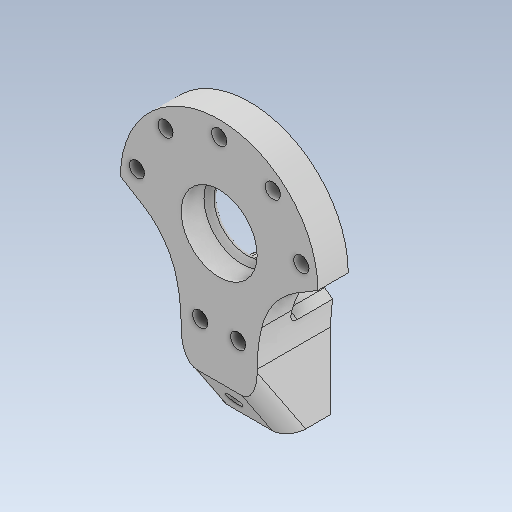
# Autodesk Inventor part: bone_upper_2
Saved by Autodesk Inventor 2020 (Build 240168000, 168)
## iProperties
Created: 2019-05-04
Part Number: bone_upper_2
Material: Generic
Document SubType Name: Modeling
Designer: psrob
Density: 1 g/cm^3
Appearance: Default
Author: psrob
Autodesk Inventor part; units mm, degrees
ref_plane "YZ Plane" through (0, 0, 0) normal (1, 0, 0) x (0, 1, 0)
ref_plane "XZ Plane" through (0, 0, 0) normal (0, 1, 0) x (-1, 0, 0)
ref_plane "XY Plane" through (0, 0, 0) normal (0, 0, 1) x (1, 0, 0)
sketch "Sketch1" plane through (0, 0, 0) normal (0, 0, 1) x (1, 0, 0)
  line L0 (0, 50) -> (6, 50) projected
  circle A0 centre (3, -17) radius 2 projected
  line L1 (3, -17) -> (3, 63)
  circle A1 centre (3, 63) radius 8
  line L2 (6, 50) -> (8, 50)
  line L3 (8, 50) -> (-2, 50)
  line L4 (-2, 50) -> (-2, 40)
  line L5 (-2, 40) -> (8, 40)
  line L6 (8, 40) -> (8, 50)
  line L7 (3, 63) -> (10.191, 59.4944)
  line L8 (3, 63) -> (-4.191, 59.4944)
  arc A2 (10.191, 59.4944) -> (8, 50) centre (29.6667, 50) ccw
  arc A3 (-2, 50) -> (-4.191, 59.4944) centre (-23.6667, 50) ccw
  arc A4 (10.191, 59.4944) -> (-4.191, 59.4944) centre (3, 63) ccw
  point P0 (0, 0)
  dimension "d0" = 80
  dimension "d1" = 16
  dimension "d2" = 2
  dimension "d3" = 10
  dimension "d4" = 10
  dimension "d5" = 8
  constraints: 16 end point, 8 point on circle, 4 centre point, 4 line through centre, 2 horizontal, 2 parallel, 1 coincident, 1 perpendicular, 1 vertical
  measures "d0" distance of L1.start L1.end
  measures "d1" diameter of A1
  measures "d2" distance of L0.end L2.end
  measures "d3" distance of L5.end L4.end
  measures "d4" distance of L4.end L3.end
  measures "d5" radius of A4
extrude "Extrusion1" add sketch "Sketch1" along normal blind 10 contours L3 A3 A1 L1 L0 | L0 L1 L5 L4 L3 | L1 A1 A2 L2 L0 | L0 L2 L6 L5 L1 | A1 L8 L1 | L1 L7 A1 | A1 L7 L8
sketch "Sketch2" plane through (0, 0, 0) normal (0, 0, -1) x (-1, 0, 0)
  arc A0 (4.191, 59.4944) -> (-10.191, 59.4944) centre (-3, 63) ccw projected
  arc A1 (-8, 50) -> (-10.191, 59.4944) centre (-29.6667, 50) ccw projected
  line L0 (-8, 40) -> (-8, 50) projected
  line L1 (2, 40) -> (-8, 40) projected
  line L2 (2, 50) -> (2, 40) projected
  arc A2 (4.191, 59.4944) -> (2, 50) centre (23.6667, 50) ccw projected
  circle A3 centre (-3, 63) radius 9
  point P0 (0, 0)
  dimension "d8" = 18
  constraints: 1 centre point, 1 coincident
  measures "d8" diameter of A3
extrude "Extrusion2" cut sketch "Sketch2" against normal blind 2.7 contours A2 A3 A1 A0 | A0 A1 A3 A2
sketch "Sketch3" plane through (0, 0, 0) normal (0, 0, -1) x (-1, 0, 0)
  arc A0 (-8.9096, 56.212) -> (2.9096, 56.212) centre (-3, 63) ccw projected
  arc A1 (-8, 50) -> (-8.9096, 56.212) centre (-29.6667, 50) ccw projected
  line L0 (-8, 40) -> (-8, 50) projected
  line L1 (2, 40) -> (-8, 40) projected
  line L2 (2, 50) -> (2, 40) projected
  arc A2 (2.9096, 56.212) -> (2, 50) centre (23.6667, 50) ccw projected
  line L3 (-6, 50) -> (0, 50) projected
  line L4 (0, 0) -> (0, 50) projected
  line L5 (-6, 0) -> (-6, 50) projected
  point P0 (-6, 40)
  point P1 (0, 40)
extrude "Extrusion3" add sketch "Sketch3" along normal blind 3 contours A0 A2 L2 L1 L4 L3 L5 L0 A1
chamfer "Chamfer1" distance 3 angle 45 4 edges at (8.9096, 56.212, -1.5) (8.9096, 56.212, 1.35) (-2.9096, 56.212, -1.5) (-2.9096, 56.212, 1.35)
fillet "Fillet1" radius 1 3 edges at (7.3004, 53.9661, 2.7) (3, 54, 2.7) (-1.3004, 53.9661, 2.7)
thicken "Thicken1" operation add thickness 3.3 both sides no extend neighbours yes toward (0, 0, -1) faces at (4.7662, 63.054, 10)
sketch "Sketch4" plane through (0, 0, -3) normal (0, 0, -1) x (-1, 0, 0)
  line L0 (0.3503, 54.6468) -> (2.2505, 53.2853) projected
  arc A0 (-6.3503, 54.6468) -> (0.3503, 54.6468) centre (-3, 63) ccw projected
  line L1 (-8.2505, 53.2853) -> (-6.3503, 54.6468) projected
  arc A1 (-8, 50) -> (-8.2505, 53.2853) centre (-29.6667, 50) ccw projected
  line L2 (-8, 50) -> (-8, 40) projected
  line L3 (-8, 40) -> (-6, 40) projected
  line L4 (-6, 40) -> (-6, 50) projected
  line L5 (-6, 50) -> (0, 50) projected
  line L6 (0, 50) -> (0, 40) projected
  line L7 (0, 40) -> (2, 40) projected
  line L8 (2, 40) -> (2, 50) projected
  arc A2 (2.2505, 53.2853) -> (2, 50) centre (23.6667, 50) ccw projected
  line L9 (-6, 50) -> (0, 50) projected
  line L10 (-3, 50) -> (-3, 52)
  line L11 (-3, 52) -> (-0.5, 52)
  line L12 (-0.5, 52) -> (-5.5, 52)
  circle A3 centre (-0.5, 52) radius 1
  circle A4 centre (-5.5, 52) radius 1
  point P0 (0, 0)
  dimension "d19" = 2
  dimension "d20" = 2.5
  dimension "d21" = 5
  dimension "d22" = 2
  dimension "d23" = 2
  constraints: 6 end point, 2 centre point, 2 coincident, 1 midpoint, 1 perpendicular, 1 point on line, 1 vertical
  measures "d19" distance of L10.start L10.end
  measures "d20" distance of L10.end L11.end
  measures "d21" distance of L11.end L12.end
  measures "d22" diameter of A3
  measures "d23" diameter of A4
extrude "Extrusion4" cut sketch "Sketch4" against normal blind 10 contours A3 | A4
sketch "Sketch5" plane through (8, 40, -3) normal (1, 0, 0) x (0, 0, -1)
  line L0 (0, 10) -> (-9.7, 10) projected
  line L1 (-9.7, 0) -> (-9.7, 10) projected
  line L2 (0, 0) -> (-9.7, 0) projected
  line L3 (0, 10) -> (0, 0) projected
  line L4 (-9.7, 0) -> (-9.7, 10) projected
  line L5 (-9.7, 0) -> (-9.7, 6)
  line L6 (-9.7, 0) -> (-5.7, 0)
  line L7 (0, 0) -> (-9.7, 0) projected
  line L8 (-9.7, 6) -> (-5.7, 0)
  point P0 (-3, -40)
  point P1 (-5.7, 0)
  dimension "d26" = 6
  dimension "d27" = 4
  constraints: 6 end point, 2 point on line
  measures "d26" distance of L1.start L5.end
  measures "d27" distance of L1.start L6.end
extrude "Extrusion5" cut sketch "Sketch5" against normal blind 10 contours L8 L2 L1
fillet "Fillet2" radius 2 2 edges at (-2, 43, 4.7) (8, 43, 4.7)
fillet "Fillet3" radius 2 6 edges at (6.3897, 54.9866, 2.4133) (6.3503, 54.6468, -1.5) (6.3503, 54.6468, 0.85) (-0.3897, 54.9863, 2.4131) (-0.3503, 54.6468, 0.85) (-0.3503, 54.6468, -1.5)
sketch "Sketch6" plane through (0, 46, 6.7) normal (0, -0.5547002, 0.8320503) x (1, 0, 0)
  line L0 (6, 0) -> (6, -7.2111) projected
  line L1 (0, 0) -> (6, 0) projected
  line L2 (0, -7.2111) -> (0, 0) projected
  line L3 (6, -7.2111) -> (0, -7.2111) projected
  line L4 (0, -7.2111) -> (6, 0)
  line L5 (6, -7.2111) -> (0, 0)
  circle A0 centre (3, -3.6056) radius 1
  point P0 (0, -41.9908)
  dimension "d32" = 2
  constraints: 4 end point, 1 centre point, 1 midpoint
  measures "d32" diameter of A0
extrude "Extrusion6" cut sketch "Sketch6" against normal blind 7 contours A0 L5 L4 | L4 L5 A0 | A0 L4 L5 | L5 L4 A0
sketch "Sketch7" plane through (3, 63, 6.7) normal (0, 0, 1) x (1, 0, 0)
  ellipse E0 centre (3, -13.3944) end of major axis (3, -17) minor radius 2 (3, -17) -> (5, -13.3944) ccw projected
  line L0 (5, -13.3944) -> (5, -13) projected
  arc A0 (7.191, -3.5056) -> (5, -13) centre (26.6667, -13) ccw projected
  arc A1 (7.191, -3.5056) -> (-7.191, -3.5056) centre (0, 0) ccw projected
  arc A2 (-5, -13) -> (-7.191, -3.5056) centre (-26.6667, -13) ccw projected
  line L1 (-5, -13) -> (-5, -13.3944) projected
  ellipse E1 centre (-3, -13.3944) end of major axis (-3, -17) minor radius 2 (-5, -13.3944) -> (-3, -17) ccw projected
  line L2 (-3, -17) -> (3, -17) projected
  circle A3 centre (-2.5, -11) radius 1 projected
  circle A4 centre (2.5, -11) radius 1 projected
  circle A5 centre (0, 0) radius 5
  point P0 (-3, -63)
  dimension "d35" = 10
  constraints: 1 centre point, 1 coincident, 2 other
  measures "d35" diameter of A5
extrude "Extrusion7" cut sketch "Sketch7" against normal blind 7 contours A5
sketch "Sketch8" plane through (0, 0, 2.7) normal (0, 0, -1) x (-1, 0, 0)
  circle A0 centre (-3, 63) radius 5 projected
  circle A1 centre (-3, 63) radius 4
  point P0 (0, 0)
  dimension "d38" = 8
  constraints: 1 centre point, 1 coincident
  measures "d38" diameter of A1
extrude "Extrusion8" add sketch "Sketch8" against normal blind 1
chamfer "Chamfer2" distance 1 angle 45 1 edges at (7, 63, 3.7)
fillet "Fillet4" radius 0.2 2 edges at (7, 63, 2.7001) (7, 63, 2.7)
sketch "Sketch12" plane through (3, 63, 6.7) normal (0, 0, 1) x (1, 0, 0)
  arc A0 (13, 0) -> (-13, 0) centre (0, 0) ccw projected
  line L0 (-13, 0) -> (-9, 0) projected
  arc A1 (9, 0) -> (-9, 0) centre (0, 0) ccw projected
  line L1 (9, 0) -> (13, 0) projected
  arc A2 (7.191, -3.5056) -> (-7.191, -3.5056) centre (0, 0) ccw projected
  line L2 (-13, 0) -> (-8, 0)
  line L3 (8, 0) -> (13, 0)
  circle A3 centre (0, 11) radius 1 projected
  circle A4 centre (7.0707, 8.4265) radius 1 projected
  circle A5 centre (-7.0707, 8.4265) radius 1 projected
  circle A6 centre (10.8329, 1.9101) radius 1 projected
  circle A7 centre (-10.8329, 1.9101) radius 1 projected
  point P0 (-3, -63)
  point P1 (9, 0)
  point P2 (-9, 0)
  constraints: 4 end point, 2 point on circle, 1 collinear, 1 horizontal, 1 point on line
extrude "Extrusion12" add sketch "Sketch12" against normal blind 4 contours L1 A1 L0 A0 | L3 A2 L2 A1 | A3 | A4 | A5 | A6 | A7
sketch "Sketch13" plane through (0, 46, 6.7) normal (0, 0, 1) x (1, 0, 0)
  circle A0 centre (3, 17) radius 5 projected
  ellipse E0 centre (6, 3.6056) end of major axis (6, 0) minor radius 2 (6, 0) -> (8, 3.6056) ccw projected
  line L0 (8, 3.6056) -> (8, 4) projected
  arc A1 (10.191, 13.4944) -> (8, 4) centre (29.6667, 4) ccw projected
  arc A2 (10.191, 13.4944) -> (11, 17) centre (3, 17) ccw projected
  line L1 (11, 17) -> (16, 17) projected
  arc A3 (16, 17) -> (-10, 17) centre (3, 17) ccw projected
  line L2 (-10, 17) -> (-5, 17) projected
  arc A4 (-5, 17) -> (-4.191, 13.4944) centre (3, 17) ccw projected
  arc A5 (-2, 4) -> (-4.191, 13.4944) centre (-23.6667, 4) ccw projected
  line L3 (-2, 4) -> (-2, 3.6056) projected
  ellipse E1 centre (0, 3.6056) end of major axis (0, 0) minor radius 2 (-2, 3.6056) -> (0, 0) ccw projected
  line L4 (0, 0) -> (6, 0) projected
  circle A6 centre (0.5, 6) radius 1 projected
  circle A7 centre (5.5, 6) radius 1 projected
  arc A8 (16, 17) -> (-10, 17) centre (3, 17) ccw projected
  line L5 (10.191, 13.4944) -> (16, 17)
  arc A9 (-5, 17) -> (-4.191, 13.4944) centre (3, 17) ccw projected
  line L6 (-4.191, 13.4944) -> (-10, 17)
  point P0 (0, -46)
  constraints: 4 end point, 2 other
extrude "Extrusion13" add sketch "Sketch13" against normal blind 4 contours A2 L1 L5 | L6 L2 A4
fillet "Fillet6" radius 10 2 edges at (10.191, 59.4944, 4.7) (-4.191, 59.4944, 4.7)
sketch "Sketch14" plane through (0, 46, 6.7) normal (0, 0, 1) x (1, 0, 0)
  arc A0 (16, 17) -> (-10, 17) centre (3, 17) ccw projected
  arc A1 (12, 17) -> (-6, 17) centre (3, 17) ccw projected
  circle A2 centre (3, 17) radius 4.4828 projected
  line L0 (3, 17) -> (3, 28)
  circle A3 centre (3, 28) radius 1
  circle A4 centre (-4.0707, 25.4265) radius 1
  circle A5 centre (-7.8329, 18.9101) radius 1
  circle A6 centre (10.0707, 25.4265) radius 1
  circle A7 centre (13.8329, 18.9101) radius 1
  point P0 (0, -46)
  dimension "d67" = 11
  dimension "d68" = 2
  dimension "d71" = 80
  dimension "d75" = 80
  constraints: 5 centre point, 2 coincident, 2 end point, 1 vertical, 11 other
  measures "d67" distance of L0.start L0.end
  measures "d68" diameter of A3
extrude "Extrusion14" cut sketch "Sketch14" against normal blind 4 contours A3 | A4 | A5 | A6 | A7
body "Solid1"
